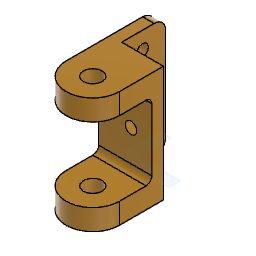
cad2 project (Autodesk Fusion 360 design; units mm, degrees)
Autodesk Fusion 360 part; units mm, degrees
sketch "Sketch1" plane through (0, 0, 0) normal (1, 0, 0) x (0, 1, 0)
  line L0 (31, 65) -> (59, 65)
  line L1 (69, 55) -> (69, -25)
  line L2 (59, -35) -> (31, -35)
  line L3 (31, -35) -> (31, 65)
  arc A0 (69, 55) -> (59, 65) centre (59, 55) ccw
  arc A1 (59, -35) -> (69, -25) centre (59, -25) ccw
  circle A2 centre (49, 49.8877) radius 5
  line L4 (31, -35) -> (31, -20)
  circle A3 centre (49, -20) radius 5
  point P0 (69, 65)
  point P1 (69, -35)
  point P2 (50, 15)
  dimension "d1" = 38
  dimension "d2" = 100
  dimension "d3" = 10
  dimension "d4" = 10
  dimension "d9" = 10
  dimension "d12" = 10
  constraint coincident P0 L0
  constraint coincident P0 L1
  constraint coincident P1 L2
  constraint coincident P1 L1
  constraint perpendicular L2 L4
  measures "d1" distance of P1 L2.end
  measures "d2" distance of P0 P1
  measures "d3" radius of A0
  measures "d4" radius of A1
  measures "d9" diameter of A2
  measures "d12" diameter of A3
extrude "Extrude1" add sketch "Sketch1" against normal blind 10
sketch "Sketch2" plane through (0, 0, 0) normal (0, 1, 0) x (1, 0, 0)
sketch "Sketch3" plane through (0, 0, 0) normal (0, 1, 0) x (1, 0, 0)
sketch "Sketch4" plane through (0, 31, 0) normal (0, -1, 0) x (1, 0, 0)
  line L0 (0, -35) -> (0, 65)
  line L1 (0, 65) -> (-10, 65)
  line L2 (-10, 65) -> (-10, -35)
  line L3 (-10, -35) -> (0, -35)
  line L4 (-10, 65) -> (36, 65)
  line L5 (36, 65) -> (36, -35)
  line L6 (36, -35) -> (-10, -35)
  dimension "d19" = 46
  constraint coincident L1.end L2.start
  constraint perpendicular L0 L4
  constraint perpendicular L4 L5
  constraint coincident L2.end L3.start
  constraint perpendicular L2 L6
  measures "d19" distance of L1.end L4.end
extrude "Extrude2" add sketch "Sketch4" along normal blind 10 contours L0 L4 L5 L6
extrude "Extrude3" add 1 faces at (-3.3333, 31, 31.6667) along direction (0, -1, 0) blind 10
sketch "Sketch5" plane through (0, 21, 0) normal (0, -1, 0) x (1, 0, 0)
  line L0 (36, -35) -> (36, 65)
  line L1 (36, 65) -> (-10, 65)
  line L2 (-10, 65) -> (-10, -35)
  line L3 (-10, -35) -> (36, -35)
  circle A0 centre (18, 15) radius 5
  dimension "d24" = 10
  measures "d24" diameter of A0
extrude "Extrude4" cut sketch "Sketch5" against normal through all contours A0
sketch "Sketch6" plane through (0, 0, 65) normal (0, 0, 1) x (-1, 0, 0)
  line L0 (0, -31) -> (0, -59)
  line L1 (0, -59) -> (10, -59)
  line L2 (10, -59) -> (10, -21)
  line L3 (10, -21) -> (-36, -21)
  line L4 (-36, -21) -> (-36, -31)
  line L5 (-36, -31) -> (0, -31)
  line L6 (10, -21) -> (10, 7)
  line L7 (-36, -21) -> (-36, 7)
  arc A0 (10, 7) -> (-36, 7) centre (-13, 7) ccw
  circle A1 centre (-13, 7) radius 8
  dimension "d40" = 16
  constraint coincident L2.end L3.start
  constraint perpendicular L3 L6
  constraint coincident L3.end L4.start
  constraint perpendicular L3 L7
  constraint tangent L6 A0
  constraint concentric A0 A1
  measures "d40" diameter of A1
extrude "Extrude5" add sketch "Sketch6" against normal blind 18 contours L3 L6 L7 A0
fillet "Fillet1" radius 5 1 edges at (13, 21, 47)
sketch "Sketch7" plane through (0, 0, 0) normal (0, 0, 1) x (1, 0, 0)
sketch "Sketch8" plane through (0, 0, -35) normal (0, 0, -1) x (1, 0, 0)
  line L0 (0, -59) -> (0, -31)
  line L1 (0, -31) -> (36, -31)
  line L2 (36, -31) -> (36, -21)
  line L3 (36, -21) -> (-10, -21)
  line L4 (-10, -21) -> (-10, -59)
  line L5 (-10, -59) -> (0, -59)
sketch "Sketch9" plane through (0, 0, -35) normal (0, 0, -1) x (1, 0, 0)
sketch "Sketch10" plane through (0, 0, -35) normal (0, 0, -1) x (1, 0, 0)
sketch "Sketch11" plane through (0, 0, -35) normal (0, 0, -1) x (1, 0, 0)
sketch "Sketch12" plane through (0, 0, 0) normal (0, 0, 1) x (1, 0, 0)
sketch "Sketch13" plane through (0, 0, -35) normal (0, 0, -1) x (1, 0, 0)
move_body "Move1" bodies 1 to x (1, 0, 0) y (0, 1, 0) z (0, 0, 1) at (-7.7879, -7.1503, -14.6351)
sketch "Sketch14" plane through (0, 0, -49.6351) normal (0, 0, -1) x (1, 0, 0)
  line L0 (-7.7879, -51.8497) -> (-7.7879, -23.8497)
  line L1 (-7.7879, -23.8497) -> (28.2121, -23.8497)
  line L2 (28.2121, -23.8497) -> (28.2121, -13.8497)
  line L3 (28.2121, -13.8497) -> (-17.7879, -13.8497)
  line L4 (-17.7879, -13.8497) -> (-17.7879, -51.8497)
  line L5 (-17.7879, -51.8497) -> (-7.7879, -51.8497)
  line L6 (-17.7879, -13.8497) -> (-17.7879, 14.1503)
  line L7 (28.2121, -13.8497) -> (28.2121, 14.1503)
  arc A0 (28.2121, 14.1503) -> (-17.7879, 14.1503) centre (5.2121, 14.1503) ccw
  circle A1 centre (5.2121, 14.1503) radius 8
  dimension "d52" = 28
  dimension "d54" = 16
  constraint coincident L3.end L4.start
  constraint perpendicular L3 L6
  constraint coincident L2.end L3.start
  constraint perpendicular L3 L7
  constraint tangent L6 A0
  constraint concentric A0 A1
  measures "d52" distance of L3.end L6.end
  measures "d54" diameter of A1
extrude "Extrude6" add sketch "Sketch14" against normal blind 18 contours L3 L6 L7 A0
fillet "Fillet2" radius 5 1 edges at (5.2121, 13.8497, -31.6351)
